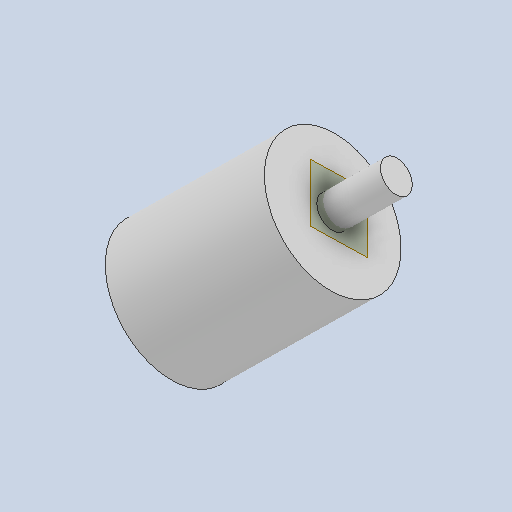
# Autodesk Inventor part: motor
Saved by Autodesk Inventor 2022 (Build 260153000, 153)
## iProperties
Created: 2022-03-03
Part Number: motor
Material: Generic
Document SubType Name: Modeling
Designer: katha
Density: 1 g/cm^3
Appearance: Default
Author: katha
Autodesk Inventor part; units mm, degrees
ref_plane "YZ Plane" through (0, 0, 0) normal (1, 0, 0) x (0, 1, 0)
ref_plane "XZ Plane" through (0, 0, 0) normal (0, 1, 0) x (-1, 0, 0)
ref_plane "XY Plane" through (0, 0, 0) normal (0, 0, 1) x (1, 0, 0)
ref_plane "Work Plane1" through (102.5092, 2.0058, -30.972) normal (-0.6788674, -0.6655937, 0.3100388) x (-0.3320481, 0.6548917, 0.6788674)
sketch "Sketch1" plane through (102.5092, 2.0058, -30.972) normal (-0.6788674, -0.6655937, 0.3100388) x (-0.3320481, 0.6548917, 0.6788674)
  circle A0 centre (0, 0) radius 2.45
  point P0 (53.7502, 45.7997)
  dimension "d0" = 4.9
  constraints: 1 centre point
  measures "d0" diameter of A0
extrude "Extrusion1" add sketch "Sketch1" along normal blind 1 and the other way blind 9
sketch "Sketch2" plane through (101.8303, 1.3402, -30.6619) normal (-0.6788674, -0.6655937, 0.3100388) x (0.4154267, 0, 0.9096267)
  circle A0 centre (0, 0) radius 2.45 projected
  circle A1 centre (0, 0) radius 10.5
  point P0 (-14.4121, 69.1303)
  dimension "d5" = 21
  constraints: 1 centre point, 1 coincident
  measures "d5" diameter of A1
extrude "Extrusion2" add sketch "Sketch2" along normal blind 25 contours A0 | A1
body "Solid1"
